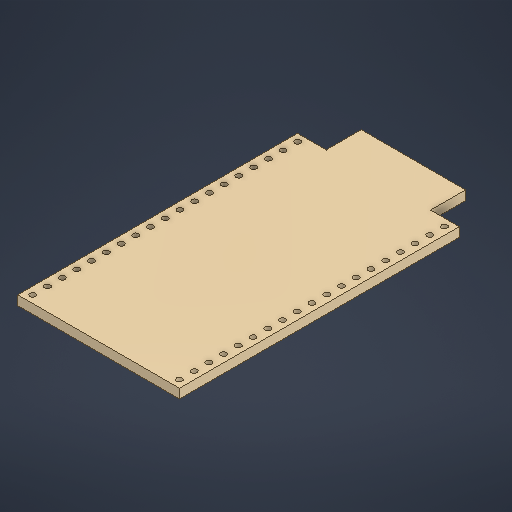
# Autodesk Inventor part: esp32-devkitc-v4
Saved by Autodesk Inventor 2025.2 (Build 292293000, 293)
## iProperties
Created: 2025-11-15
Part Number: esp32-devkitc-v4
Material: Fiberglass Batt
Document SubType Name: Modeling
Designer: sam
Density: 0.032 g/cm^3
Appearance: Golden Sand
Author: sam
Autodesk Inventor part; units mm, degrees
ref_plane "YZ Plane" through (0, 0, 0) normal (1, 0, 0) x (0, 1, 0)
ref_plane "XZ Plane" through (0, 0, 0) normal (0, 1, 0) x (-1, 0, 0)
ref_plane "XY Plane" through (0, 0, 0) normal (0, 0, 1) x (1, 0, 0)
sketch "Sketch1" plane through (0, 0, 0) normal (0, 1, 0) x (-1, 0, 0)
  line L0 (13.95, -24.13) -> (-13.95, -24.13)
  line L1 (-13.95, -24.13) -> (-13.95, 24.13)
  line L2 (-13.95, 24.13) -> (13.95, 24.13)
  line L3 (13.95, 24.13) -> (13.95, -24.13)
  line L4 (13.95, -24.13) -> (-13.95, 24.13) construction
  line L5 (-13.95, -24.13) -> (13.95, 24.13) construction
  line L6 (9, -24.13) -> (-9, -24.13)
  line L7 (-9, -24.13) -> (-9, -30.17)
  line L8 (-9, -30.17) -> (9, -30.17)
  line L9 (9, -30.17) -> (9, -24.13)
  circle A0 centre (12.65, 22.84) radius 0.5
  circle A1 centre (12.65, 20.3) radius 0.5
  circle A2 centre (12.65, 17.76) radius 0.5
  circle A3 centre (12.65, 15.22) radius 0.5
  circle A4 centre (12.65, 12.68) radius 0.5
  circle A5 centre (12.65, 10.14) radius 0.5
  circle A6 centre (12.65, 7.6) radius 0.5
  circle A7 centre (12.65, 5.06) radius 0.5
  circle A8 centre (12.65, 2.52) radius 0.5
  circle A9 centre (12.65, -0.02) radius 0.5
  circle A10 centre (12.65, -2.56) radius 0.5
  circle A11 centre (12.65, -5.1) radius 0.5
  circle A12 centre (12.65, -7.64) radius 0.5
  circle A13 centre (12.65, -10.18) radius 0.5
  circle A14 centre (12.65, -12.72) radius 0.5
  circle A15 centre (12.65, -15.26) radius 0.5
  circle A16 centre (12.65, -17.8) radius 0.5
  circle A17 centre (12.65, -20.34) radius 0.5
  circle A18 centre (12.65, -22.88) radius 0.5
  circle A19 centre (-12.65, 22.84) radius 0.5
  circle A20 centre (-12.65, 20.3) radius 0.5
  circle A21 centre (-12.65, 17.76) radius 0.5
  circle A22 centre (-12.65, 15.22) radius 0.5
  circle A23 centre (-12.65, 12.68) radius 0.5
  circle A24 centre (-12.65, 10.14) radius 0.5
  circle A25 centre (-12.65, 7.6) radius 0.5
  circle A26 centre (-12.65, 5.06) radius 0.5
  circle A27 centre (-12.65, 2.52) radius 0.5
  circle A28 centre (-12.65, -0.02) radius 0.5
  circle A29 centre (-12.65, -2.56) radius 0.5
  circle A30 centre (-12.65, -5.1) radius 0.5
  circle A31 centre (-12.65, -7.64) radius 0.5
  circle A32 centre (-12.65, -10.18) radius 0.5
  circle A33 centre (-12.65, -12.72) radius 0.5
  circle A34 centre (-12.65, -15.26) radius 0.5
  circle A35 centre (-12.65, -17.8) radius 0.5
  circle A36 centre (-12.65, -20.34) radius 0.5
  circle A37 centre (-12.65, -22.88) radius 0.5
  point P0 (0, 0)
  dimension "d6" = 27.9
  dimension "d7" = 48.26
  dimension "d8" = 18
  dimension "d9" = 6.04
  dimension "d10" = 9
  dimension "d11" = 1
  dimension "d12" = 1.29
  dimension "d13" = 1.3
  dimension "d16" = 2.54
  dimension "d21" = 1
  dimension "d22" = 1.29
  dimension "d23" = 1.3
  dimension "d26" = 2.54
  constraints: 38 centre point, 20 end point, 4 parallel, 2 horizontal, 2 midpoint, 2 perpendicular, 2 vertical, 1 point on line, 72 other
  measures "d6" distance of L1.end L2.end
  measures "d7" distance of L0.end L1.end
  measures "d8" distance of L8.end L7.end
  measures "d9" distance of L7.end L6.end
  measures "d10" distance from line of point (0, 0) L9
  measures "d11" diameter of A0
  measures "d12" distance from line of L2 A0.centre
  measures "d13" distance from line of L3 A0.centre
  measures "d16" distance of A0.centre A1.centre
  measures "d21" diameter of A19
  measures "d22" distance from line of L2 A19.centre
  measures "d23" distance from line of L1 A19.centre
  measures "d26" distance of A19.centre A20.centre
extrude "Extrusion1" add sketch "Sketch1" along normal blind 1.6
body "Solid1"
